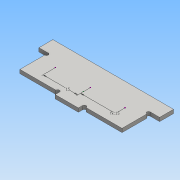
# Autodesk Inventor part: AK-C-C10-Insert-Board
Saved by Autodesk Inventor 2016 (Build 200138000, 138)
## iProperties
Created: 2016-03-31
Part Number: AK-C-C10-Insert-Board
Material: Generic
Document SubType Name: Modeling
Designer: admin
Density: 1 g/cm^3
Appearance: Default
Author: admin
Autodesk Inventor part; units mm, degrees
ref_plane "YZ Plane" through (0, 0, 0) normal (1, 0, 0) x (0, 1, 0)
ref_plane "XZ Plane" through (0, 0, 0) normal (0, 1, 0) x (-1, 0, 0)
ref_plane "XY Plane" through (0, 0, 0) normal (0, 0, 1) x (1, 0, 0)
sketch "Sketch1" plane through (0, 0, 0) normal (0, 0, 1) x (1, 0, 0)
  line L0 (-26, 12.85) -> (26, 12.85)
  line L1 (26, 12.85) -> (26, 6.85)
  line L2 (5, -7.15) -> (-5, -7.15)
  line L3 (-26, 6.85) -> (-26, 12.85)
  line L4 (-22, -5.35) -> (-22, 5.35)
  line L5 (22, -5.35) -> (22, 5.35)
  line L6 (-22, 6.85) -> (-26, 6.85)
  line L7 (22, 6.85) -> (26, 6.85)
  line L8 (0, 5.6029) -> (0, -5.6029) construction
  arc A0 (-22, 5.35) -> (-22, 6.85) centre (-22, 6.1) ccw
  arc A1 (22, 6.85) -> (22, 5.35) centre (22, 6.1) ccw
  line L9 (-5, -7.15) -> (-5, -5.35)
  line L10 (-6.5, -5.35) -> (-22, -5.35)
  line L11 (5, -7.15) -> (5, -5.35)
  line L12 (6.5, -5.35) -> (22, -5.35)
  arc A2 (-5, -5.35) -> (-6.5, -5.35) centre (-5.75, -5.35) ccw
  arc A3 (6.5, -5.35) -> (5, -5.35) centre (5.75, -5.35) ccw
  point P0 (0, 0)
  point P1 (0, 12.85)
  point P2 (26, 0)
  point P3 (0, 0)
  point P4 (-22, 0)
  dimension "d0" = 52
  dimension "d4" = 44
  dimension "d6" = 20
  dimension "d7" = 6
  dimension "d8" = 1.5
  dimension "d18" = 10
  dimension "d19" = 1.8
  dimension "d20" = 1.5
  constraints: 26 end point, 8 point on circle, 7 point on line, 4 centre point, 4 perpendicular, 4 tangent, 3 midpoint, 3 vertical, 2 equal radius, 2 horizontal, 2 horizontal alignment, 2 parallel, 1 coincident, 1 collinear, 1 vertical alignment, 2 other
  measures "d0" distance of L0.start L0.end
  measures "d4" distance between parallel lines of L5 L4
  measures "d6" distance between parallel lines of L2 L0
  measures "d7" distance between parallel lines of L6 L0
  measures "d8" diameter of A0
  measures "d18" distance of L2.start L2.end
  measures "d19" distance between parallel lines of L12 L2
  measures "d20" diameter of A2
extrude "Extrusion1" add sketch "Sketch1" along normal blind 1.6
sketch "Sketch2" plane through (0, 0, 1.6) normal (0, 0, 1) x (1, 0, 0)
  point P0 (0, 0)
  point P1 (-15, 2.97)
  point P2 (0, 2.97)
  point P3 (15, 2.97)
  dimension "d9" = 15
  dimension "d10" = 15
  constraints: 2 horizontal alignment, 1 vertical alignment
  measures "d9" distance of point (0, 2.97) point (-15, 2.97)
  measures "d10" distance of point (15, 2.97) point (0, 2.97)
equation "\"d10\" = d9"
body "Solid1"
